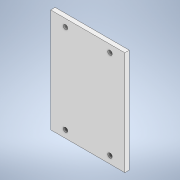
# Autodesk Inventor part: bracket-temporary-1
Saved by Autodesk Inventor 2021 (Build 250183000, 183)
## iProperties
Created: 2024-04-05
Part Number: bracket-temporary-1
Material: PC/ABS Plastic
Document SubType Name: Modeling
Designer: ASUS
Density: 0.357273 g/cm^3
Appearance: White
Author: ASUS
Autodesk Inventor part; units mm, degrees
ref_plane "YZ Plane" through (0, 0, 0) normal (1, 0, 0) x (0, 1, 0)
ref_plane "XZ Plane" through (0, 0, 0) normal (0, 1, 0) x (-1, 0, 0)
ref_plane "XY Plane" through (0, 0, 0) normal (0, 0, 1) x (1, 0, 0)
sketch "Sketch1" plane through (0, 0, 0) normal (0, 0, 1) x (1, 0, 0)
  line L0 (0, 0) -> (50, 0)
  line L1 (50, 0) -> (50, 70)
  line L2 (50, 70) -> (0, 70)
  line L3 (0, 70) -> (0, 0)
  circle A0 centre (10, 5) radius 1.5
  circle A1 centre (40, 5) radius 1.5
  circle A2 centre (10, 65) radius 1.5
  circle A3 centre (40, 65) radius 1.5
  dimension "d0" = 70
  dimension "d1" = 50
  dimension "d4" = 3
  dimension "d5" = 3
  dimension "d6" = 3
  dimension "d7" = 3
  dimension "d8" = 5
  dimension "d9" = 5
  dimension "d10" = 10
  dimension "d11" = 10
  dimension "d12" = 10
  dimension "d13" = 5
  dimension "d14" = 10
  dimension "d15" = 5
  constraints: 8 end point, 4 centre point, 2 parallel, 1 horizontal, 1 perpendicular
  measures "d0" distance between parallel lines of L0 L2
  measures "d1" distance between parallel lines of L1 L3
  measures "d4" diameter of A0
  measures "d5" diameter of A1
  measures "d6" diameter of A2
  measures "d7" diameter of A3
  measures "d8" distance from line of L0 A0.centre
  measures "d9" distance from line of L0 A1.centre
  measures "d10" distance from line of L3 A0.centre
  measures "d11" distance from line of L1 A1.centre
  measures "d12" distance from line of L3 A2.centre
  measures "d13" distance from line of L2 A2.centre
  measures "d14" distance from line of L1 A3.centre
  measures "d15" distance from line of L2 A3.centre
extrude "Extrusion1" add sketch "Sketch1" along normal blind 3
body "Solid1"
